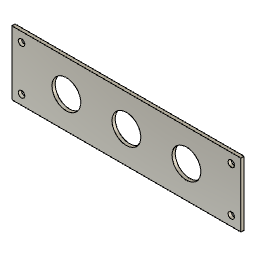
3 hole plate (Autodesk Fusion 360 design; units mm, degrees)
Autodesk Fusion 360 part; units mm, degrees
sketch "Sketch1" plane through (0, 0, 0) normal (0, 1, 0) x (1, 0, 0)
  line L0 (0, 0) -> (0, -50.0731) construction
  line L1 (-71.5, 0) -> (71.5, 0)
  line L2 (71.5, 0) -> (71.5, -40)
  line L3 (71.5, -40) -> (-71.5, -40)
  line L4 (-71.5, -40) -> (-71.5, 0)
  line L5 (-71.5, -20) -> (71.5, -20) construction
  line L6 (-65.5, -34) -> (65.5, -34) construction
  line L7 (65.5, -34) -> (65.5, -6) construction
  line L8 (65.5, -6) -> (-65.5, -6) construction
  line L9 (-65.5, -6) -> (-65.5, -34) construction
  circle A0 centre (-65.5, -34) radius 2
  circle A1 centre (65.5, -34) radius 2
  circle A2 centre (65.5, -6) radius 2
  circle A3 centre (-65.5, -6) radius 2
  circle A4 centre (37.5, -20) radius 9
  circle A5 centre (-37.5, -20) radius 9
  circle A6 centre (0, -20) radius 9
  dimension "d1" = 143
  dimension "d2" = 40
  dimension "d3" = 71.5
  dimension "d4" = 40
  dimension "d5" = 6
  dimension "d6" = 6
  dimension "d7" = 6
  dimension "d8" = 6
  dimension "d9" = 4
  dimension "d10" = 4
  dimension "d11" = 4
  dimension "d12" = 4
  dimension "d16" = 18
  dimension "d17" = 18
  dimension "d25" = 18
  dimension "d26" = 37.5
  dimension "d27" = 37.5
  constraint coincident L0.start origin
  constraint vertical L0
  constraint horizontal L1
  constraint vertical L2
  constraint horizontal L3
  constraint vertical L4
  constraint midpoint L4 L5.start
  constraint midpoint L2 L5.end
  constraint horizontal L6
  constraint vertical L7
  constraint horizontal L8
  constraint vertical L9
  constraint coincident L6.start L9.end
  constraint coincident L6.end L7.start
  constraint coincident L7.end L8.start
  constraint coincident L8.end L9.start
  constraint coincident L5 A4.centre
  constraint coincident L5 A5.centre
  constraint midpoint L5 A6.centre
  measures "d1" distance of L1.start L1.end
  measures "d2" distance of L1.start L3.end
  measures "d3" distance of L0 L2
  measures "d4" distance of L0.start L3
  measures "d5" distance of L3 L6
  measures "d6" distance of L1 L8
  measures "d7" distance of L2 L7
  measures "d8" distance of L4 L9
  measures "d9" diameter of A0
  measures "d10" diameter of A1
  measures "d11" diameter of A2
  measures "d12" diameter of A3
  measures "d16" diameter of A4
  measures "d17" diameter of A5
  measures "d25" diameter of A6
  measures "d26" distance of A5.centre A6.centre
  measures "d27" distance of A4.centre A6.centre
extrude "Extrude1" add sketch "Sketch1" along normal blind 2
equation "d3 = d1 / 2"
equation "d4 = d2"
equation "d6 = d5"
equation "d8 = d7"
equation "d10 = d9"
equation "d11 = d9"
equation "d12 = d9"
equation "HoleSpread = 75 mm"
equation "HoleDia = 18 mm"
equation "d16 = HoleDia"
equation "d17 = HoleDia"
equation "d25 = HoleDia"
equation "d26 = HoleSpread / 2"
equation "d27 = HoleSpread / 2"
named bodies: "Panel"
